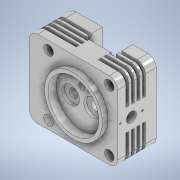
# Autodesk Inventor part: Peça5
Saved by Autodesk Inventor 2021 (Build 250183000, 183)
## iProperties
Created: 2021-07-18
Part Number: Peça5
Material: Alumínio 6061
Document SubType Name: Modeling
Designer: Giovanni
Density: 2.7 g/cm^3
Appearance: Alumínio - Polido
Author: Giovanni
Autodesk Inventor part; units mm, degrees
ref_plane "YZ Plane" through (0, 0, 0) normal (1, 0, 0) x (0, 1, 0)
sketch "Esboço1" plane through (0, 0, 0) normal (0, 0, 1) x (1, 0, 0)
  line L0 (-75, 70) -> (55, 70)
  line L1 (70, 55) -> (70, -55)
  line L2 (55, -70) -> (-75, -70)
  line L3 (-90, -55) -> (-90, 55)
  arc A0 (-75, 70) -> (-90, 55) centre (-75, 55) ccw
  arc A1 (70, 55) -> (55, 70) centre (55, 55) ccw
  arc A2 (55, -70) -> (70, -55) centre (55, -55) ccw
  arc A3 (-90, -55) -> (-75, -70) centre (-75, -55) ccw
  point P0 (0, 0)
  point P1 (70, -70)
  point P2 (70, 70)
  point P3 (-90, -70)
  point P4 (70, 0)
  dimension "d0" = 140
  dimension "d1" = 160
  dimension "d2" = 70
  dimension "d3" = 15
  constraints: 8 end point, 8 point on circle, 8 tangent, 6 point on line, 4 centre point, 3 equal radius, 2 parallel, 1 horizontal, 1 horizontal alignment, 1 midpoint, 1 perpendicular
  measures "d0" distance of point (70, 70) point (70, -70)
  measures "d1" distance of point (70, -70) point (-90, -70)
  measures "d2" distance from line of L1 point (0, 0)
  measures "d3" radius of A0
extrude "Extrusão1" add sketch "Esboço1" along normal blind 70
sketch "Esboço2" plane through (0, 0, 70) normal (0, 0, -1) x (-1, 0, 0)
  circle A0 centre (0, 0) radius 52.5
  dimension "d6" = 105
  constraints: 1 centre point, 1 coincident
  measures "d6" diameter of A0
extrude "Extrusão2" add sketch "Esboço2" against normal blind 10
sketch "Esboço3" plane through (0, 0, 80) normal (0, 0, 1) x (1, 0, 0)
  circle A0 centre (0, 0) radius 46
  dimension "d9" = 92
  constraints: 1 centre point, 1 coincident
  measures "d9" diameter of A0
extrude "Extrusão3" cut sketch "Esboço3" against normal blind 15
sketch "Esboço4" plane through (0, 0, 0) normal (0, 1, 0) x (-1, 0, 0)
  line L0 (75, 0) -> (-55, 0) projected
  line L1 (20, 0) -> (20, 65)
  line L2 (-46, 65) -> (46, 65) projected
  line L3 (20, 0) -> (30, 0)
  line L4 (30, 0) -> (30, 25)
  line L5 (30, 25) -> (25, 25)
  line L6 (25, 25) -> (25, 41)
  line L7 (25, 41) -> (28, 41)
  line L8 (28, 41) -> (28, 60)
  line L9 (28, 60) -> (36, 60)
  line L10 (36, 60) -> (36, 65)
  line L11 (36, 65) -> (20, 65)
  point P0 (0, 0)
  dimension "d12" = 10
  dimension "d13" = 5
  dimension "d14" = 8
  dimension "d15" = 25
  dimension "d16" = 16
  dimension "d17" = 5
  dimension "d18" = 19
  dimension "d19" = 20
  constraints: 20 end point, 4 perpendicular, 4 point on line, 2 vertical, 1 collinear
  measures "d12" distance between parallel lines of L1 L4
  measures "d13" distance between parallel lines of L1 L6
  measures "d14" distance between parallel lines of L1 L8
  measures "d15" distance of L3.end L4.end
  measures "d16" distance between parallel lines of L1 L10
  measures "d17" distance of L9.end L10.end
  measures "d18" distance of L7.end L8.end
  measures "d19" distance from line of point (0, 0) L1
revolve "Revolução1" cut sketch "Esboço4" angle 360 about axis through (-20, 0, 0) along (0, 0, 1)
mirror "Espelhamento1" about plane through (0, 0, 0) normal (1, 0, 0) of "Revolução1"
ref_plane "Plano de trabalho1" through (0, 0, 20) normal (0, 0, -1) x (-1, 0, 0)
sketch "Esboço5" plane through (0, 0, 20) normal (0, 0, -1) x (-1, 0, 0)
  line L0 (67.082, 20) -> (90, 20)
  line L1 (67.082, -20) -> (90, -20)
  line L2 (-67.082, 20) -> (-70, 20)
  line L3 (-67.082, -20) -> (-70, -20)
  line L4 (-20, 67.082) -> (-20, 70)
  line L5 (20, 67.082) -> (20, 70)
  line L6 (-20, -67.082) -> (-20, -70)
  line L7 (20, -67.082) -> (20, -70)
  arc A0 (-55, 70) -> (-70, 55) centre (-55, 55) ccw projected
  line L8 (-55, 70) -> (75, 70) projected
  arc A1 (90, 55) -> (75, 70) centre (75, 55) ccw projected
  line L9 (90, 55) -> (90, -55) projected
  arc A2 (75, -70) -> (90, -55) centre (75, -55) ccw projected
  line L10 (75, -70) -> (-55, -70) projected
  arc A3 (-70, -55) -> (-55, -70) centre (-55, -55) ccw projected
  line L11 (-70, -55) -> (-70, 55) projected
  arc A4 (67.082, 20) -> (20, 67.082) centre (0, 0) ccw
  arc A5 (-20, 67.082) -> (-67.082, 20) centre (0, 0) ccw
  arc A6 (-67.082, -20) -> (-20, -67.082) centre (0, 0) ccw
  arc A7 (20, -67.082) -> (67.082, -20) centre (0, 0) ccw
  dimension "d23" = 70
  dimension "d24" = 40
  dimension "d25" = 20
  dimension "d26" = 40
  dimension "d27" = 20
  constraints: 16 end point, 8 point on circle, 8 point on line, 4 centre point, 4 collinear, 4 horizontal, 4 vertical, 3 concentric, 1 coincident
  measures "d23" radius of A5
  measures "d24" distance between parallel lines of L1 L0
  measures "d25" distance from line of point (0, 0) L0
  measures "d26" distance of L5.end L4.end
  measures "d27" horizontal distance of point (0, 0) L4.end
extrude "Extrusão4" cut sketch "Esboço5" against normal blind 5 contours A4 L5 L8 A1 L9 L0 | L9 A2 L10 L7 A7 L1 | L4 A5 L2 L11 A0 L8 | L10 A3 L11 L3 A6 L6
pattern_linear "Padrão retangular1" count 4 spacing 10 along (0, 0, 1) of "Extrusão4"
sketch "Esboço6" plane through (0, 0, 0) normal (1, 0, 0) x (0, 1, 0)
  line L0 (70, 0) -> (70, 20) projected
  line L1 (70, 0) -> (15, 0)
  line L2 (15, 0) -> (15, 17)
  line L3 (15, 17) -> (70, 31.7372)
  line L4 (70, 31.7372) -> (70, 0)
  point P0 (0, 0)
  dimension "d33" = 55
  dimension "d34" = 17
  dimension "d35" = 15
  constraints: 8 end point, 1 horizontal, 1 vertical
  measures "d33" distance of L0.start L1.end
  measures "d34" distance of L1.end L2.end
  measures "d35" angle of L3 L1
extrude "Extrusão5" cut sketch "Esboço6" against normal mid plane 55
sketch "Esboço7" plane through (27.5, 15, 17) normal (0, 0.2588, -0.9659) x (-1, 0, 0)
  circle A0 centre (27.5, 20) radius 16
  line L0 (55, -4.3999) -> (0, -4.3999) projected
  line L1 (0, 0) -> (55, 0) projected
  point P0 (27.5, -18.8888)
  dimension "d39" = 20
  dimension "d40" = 32
  constraints: 1 centre point, 1 vertical alignment
  measures "d39" distance from line of L1 A0.centre
  measures "d40" diameter of A0
extrude "Extrusão6" cut sketch "Esboço7" against normal blind 32
sketch "Esboço8" plane through (0, 26.0363, 53.086) normal (0, 0.2588, -0.9659) x (-1, 0, 0)
  circle A0 centre (0, 0) radius 16 projected
  point P0 (0, -38.8888)
  constraints: 1 coincident
hole "Furo1" at (0, 26.0363, 53.086) direction (0, -0.2588, 0.9659) diameter 11.835 depth 40 tip angle 118 thread size "M14x2" class "6H" standard "ANSI Metric M Profile"
sketch "Esboço9" plane through (0, 0, 0) normal (0, 0, -1) x (-1, 0, 0)
  arc A0 (-70, -55) -> (-55, -70) centre (-55, -55) ccw projected
  arc A1 (-55, 70) -> (-70, 55) centre (-55, 55) ccw projected
  arc A2 (90, 55) -> (75, 70) centre (75, 55) ccw projected
  arc A3 (75, -70) -> (90, -55) centre (75, -55) ccw projected
  point P0 (0, 0)
  point P1 (55, 55)
  point P2 (55, -55)
  dimension "d50" = 55
  dimension "d51" = 55
  constraints: 2 coincident, 2 horizontal alignment
  measures "d50" horizontal distance of point (0, 0) point (55, -55)
  measures "d51" horizontal distance of point (0, 0) point (55, 55)
hole "Furo2" at (55, -55, 0) at (55, 55, 0) at (-55, 55, 0) at (-55, -55, 0) direction (0, 0, 1) diameter 17.5 end through all
sketch "Esboço10" plane through (-90, -55, 0) normal (-1, 0, 0) x (0, 0, 1)
  circle A0 centre (45, 55) radius 9
  line L0 (70, 110) -> (70, 0) projected
  point P0 (0, 55)
  point P1 (70, 55)
  dimension "d59" = 18
  dimension "d60" = 25
  constraints: 1 centre point, 1 horizontal alignment, 1 midpoint
  measures "d59" diameter of A0
  measures "d60" distance from line of L0 A0.centre
extrude "Extrusão7" cut sketch "Esboço10" against normal blind 10
sketch "Esboço11" plane through (-80, 0, 45) normal (-1, 0, 0) x (0, 0, 1)
  circle A0 centre (0, 0) radius 9 projected
  point P0 (-45, 0)
  constraints: 1 coincident
hole "Furo3" at (-80, 0, 45) direction (1, 0, 0) diameter 8 depth 60
sketch "Esboço12" plane through (-90, -55, 0) normal (-1, 0, 0) x (0, 0, 1)
  circle A0 centre (45, 55) radius 4 projected
  point P0 (0, 55)
  point P1 (25, 55)
  point P2 (65, 55)
  dimension "d70" = 20
  dimension "d72" = 20
  constraints: 2 horizontal alignment
  measures "d70" distance of A0.centre point (25, 55)
  measures "d72" distance of A0.centre point (65, 55)
hole "Furo4" at (-90, 0, 25) at (-90, 0, 65) direction (1, 0, 0) diameter 3.242 depth 15 tip angle 118 thread size "M4x0.7" class "6H" standard "ANSI Metric M Profile"
ref_plane "Plano de trabalho2" through (-10, -55, 0) normal (1, 0, 0) x (0, 0, -1)
mirror "Espelhamento2" about plane through (-10, -55, 0) normal (1, 0, 0) of "Extrusão7", "Furo3", "Furo4"
sketch "Esboço13" plane through (0, 0, 0) normal (0, 0, -1) x (-1, 0, 0)
  line L0 (75, -70) -> (-55, -70) projected
  point P0 (0, 0)
  point P1 (20, -57)
  point P2 (-20, -57)
  dimension "d80" = 20
  dimension "d81" = 20
  dimension "d82" = 13
  constraints: 1 horizontal alignment
  measures "d80" horizontal distance of point (0, 0) point (20, -57)
  measures "d81" horizontal distance of point (-20, -57) point (0, 0)
  measures "d82" distance from line of L0 point (-20, -57)
hole "Furo5" at (-20, -57, 0) at (20, -57, 0) direction (0, 0, 1) diameter 3.242 depth 15 tip angle 118 thread size "M4x0.7" class "6H" standard "ANSI Metric M Profile"
